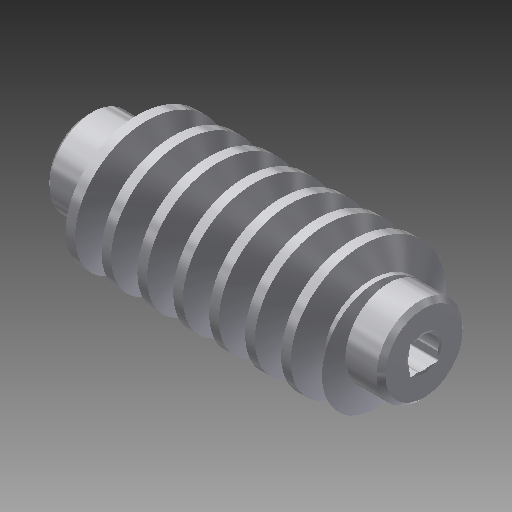
# Autodesk Inventor part: 400-04
Saved by Autodesk Inventor 2019 (Build 230136000, 136)
## iProperties
Created: 2007-11-19
Part Number: 400-04
Material: Acetal Resin, White
Document SubType Name: Modeling
Designer: Autodesk Inc.
Density: 1.425 g/cm^3
Mass: 5.8548 g
Surface Area: 32.563 cm^2
Volume: 4.10863 cm^3
Description: WORM GEAR
Appearance: Smooth - White
CustomPartVersion: 1
Company: Autodesk Inc.
Component Category: Lower Component
d49: 20.000 mm
d50: 0.000 mm
d54: 0.000 mm
d56: 0.000 mm
d77: 0.000 mm
d79: 20.000 mm
d80: 0.000 mm
Author: Inventor
Autodesk Inventor part; units mm, degrees
ref_plane "YZ Plane" through (0, 0, 0) normal (1, 0, 0) x (0, 1, 0)
ref_plane "XZ Plane" through (0, 0, 0) normal (0, 1, 0) x (-1, 0, 0)
ref_plane "XY Plane" through (0, 0, 0) normal (0, 0, 1) x (1, 0, 0)
sketch "Base Body Sketch" plane through (0, 0, 0) normal (1, 0, 0) x (0, 1, 0)
  circle A0 centre (0, 0) radius 7.761668
  dimension "d5" = 15.52334
extrude "Base Body" add sketch "Base Body Sketch" along normal mid plane 30
sketch "Sketch5" plane through (15, 0, 0) normal (1, 0, 0) x (0, 0, -1)
  circle A0 centre (0, 0) radius 7.761668
  circle A1 centre (0, 0) radius 6.5
  dimension "d59" = 13
  constraints: 1 centre point, 1 coincident
  measures "d59" diameter of A1
sketch "Sketch7" plane through (0, 0, 0) normal (0, 1, 0) x (-1, 0, 0)
  line L0 (13.658997, -4.915723) -> (12.757003, -4.915723)
  line L1 (11.721164, -7.761668) -> (10.630836, -7.761668)
  line L2 (9.594997, -4.915723) -> (8.693003, -4.915723)
  line L3 (7.657164, -7.761668) -> (6.566836, -7.761668)
  line L4 (5.530997, -4.915723) -> (4.629003, -4.915723)
  line L5 (3.593164, -7.761668) -> (2.502836, -7.761668)
  line L6 (1.466997, -4.915723) -> (0.565003, -4.915723)
  line L7 (-0.470836, -7.761668) -> (-1.561164, -7.761668)
  line L8 (-2.597003, -4.915723) -> (-3.498997, -4.915723)
  line L9 (15, 4.915723) -> (15, 4.865723)
  line L10 (15, 4.865723) -> (18.5, 4.865723)
  line L11 (18.5, 4.865723) -> (19, 4.365723)
  line L12 (19, 4.365723) -> (19, -4.365723)
  line L13 (19, -4.365723) -> (18.5, -4.865723)
  line L14 (18.5, -4.865723) -> (15, -4.865723)
  line L15 (15, -4.865723) -> (15, -4.915723)
  line L16 (19, 0) -> (27, 0) construction
  arc A0 (19, 2.015564) -> (18.75, 0) centre (27, 0) ccw
  line L17 (19, 0) -> (18.75, 0)
  line L18 (19, 0) -> (19, 2.015564)
  line L19 (15, -4.915723) -> (14.329498, -6.757911)
  line L20 (-15, 4.915723) -> (-14.329498, 6.757911)
  line L21 (-4.534836, -7.761668) -> (-5.625164, -7.761668)
  line L22 (-11.721164, 7.761668) -> (-10.630836, 7.761668)
  line L23 (-13.658997, 4.915723) -> (-12.757003, 4.915723)
  line L24 (-7.657164, 7.761668) -> (-6.566836, 7.761668)
  line L25 (-9.594997, 4.915723) -> (-8.693003, 4.915723)
  line L26 (14.789003, 4.915723) -> (15, 4.915723)
  line L27 (-6.661003, -4.915723) -> (-7.562997, -4.915723)
  line L28 (-8.598836, -7.761668) -> (-9.689164, -7.761668)
  line L29 (-10.725003, -4.915723) -> (-11.626997, -4.915723)
  line L30 (-12.662836, -7.761668) -> (-13.753164, -7.761668)
  line L31 (-14.789003, -4.915723) -> (-15, -4.915723)
  line L32 (-15, -4.915723) -> (-15, 4.915723)
  line L33 (-5.530997, 4.915723) -> (-4.629003, 4.915723)
  line L34 (-3.593164, 7.761668) -> (-2.502836, 7.761668)
  line L35 (-1.466997, 4.915723) -> (-0.565003, 4.915723)
  line L36 (0.470836, 7.761668) -> (1.561164, 7.761668)
  line L37 (2.597003, 4.915723) -> (3.498997, 4.915723)
  line L38 (4.534836, 7.761668) -> (5.625164, 7.761668)
  line L39 (6.661003, 4.915723) -> (7.562997, 4.915723)
  line L40 (8.598836, 7.761668) -> (9.689164, 7.761668)
  line L41 (10.725003, 4.915723) -> (11.626997, 4.915723)
  line L42 (12.662836, 7.761668) -> (13.753164, 7.761668)
  dimension "d87" = 8
  dimension "d88" = 16.5
  constraints: 6 end point, 2 collinear, 2 point on circle, 1 centre point, 1 coincident, 1 midpoint, 1 perpendicular, 1 point on line, 30 other
  measures "d87" distance of L16.start L16.end
  measures "d88" diameter of A0
surface extrude "ExtrusionSrf1" sketch "Sketch5" against normal through all shown no curves A1
chamfer "Chamfer1" distance 1.035839 distance2 2.845945 1 edges at (15, -7.7617, 0) measured on face at (10, 7.7365, -0.6246)
chamfer "Chamfer2" distance 1.035839 distance2 2.845945 1 edges at (-15, -7.7617, 0) measured on face at (-10, 7.7365, -0.6246)
sketch "Tooth Sketch" plane through (0, 0, 0) normal (0, 0, 1) x (1, 0, 0)
  line L0 (0, 8.423997) -> (0, 4.331011)
  line L1 (-19.803086, 7.839285) -> (-18.738997, 4.915723)
  line L2 (-17.837003, 4.915723) -> (-16.772914, 7.839285)
  line L3 (-20.409121, 0) -> (-16.166879, 0)
  line L4 (-19.803086, 7.839285) -> (-18.288, 7.839285)
  line L5 (-18.288, 7.839285) -> (-16.772914, 7.839285)
  line L6 (-18.738997, 4.915723) -> (-18.288, 4.915723)
  line L7 (-18.288, 4.915723) -> (-17.837003, 4.915723)
  line L8 (-18.288, 6.468057) -> (-17.272, 6.468057) construction
  line L9 (-18.288, 7.839285) -> (-18.288, 4.915723) construction
  dimension "d24" = 110
  dimension "d25" = 18.288
  dimension "d26" = 1.016
  dimension "d27" = 4.91572
  dimension "d28" = 6.46806
  dimension "d29" = 7.83928
  constraints: 16 end point, 3 equal length, 3 parallel, 2 collinear, 2 point on line
  measures "d24" angle of L6 L1
  measures "d25" distance from line of L0 L4.end
  measures "d26" distance of L8.start L8.end
  measures "d27" distance between parallel lines of L3 L6
  measures "d28" distance between parallel lines of L3 L8
  measures "d29" distance between parallel lines of L3 L4
feature "Tooth" [suppressed]
pattern_circular "Tooth Pattern" [suppressed]
coil "Left Tooth" sketch "Tooth Sketch" operation cut axis through (-10, 0, 0) along (1, 0, 0) pitch 4.064 turns 10 hand left
pattern_of_one "Left Tooth Pattern"
sketch "Sketch6" plane through (-15, 0, 0) normal (-1, 0, 0) x (0, 0, 1)
  arc A0 (4.65648, -1.575285) -> (2.36739, 4.308109) centre (0, 0) ccw
  circle A1 centre (0, 0) radius 4.865723
  arc A2 (2.36739, 4.308109) -> (4.65648, -1.575285) centre (0, 0) ccw
  dimension "d83" = 0.05
  constraints: 1 centre point, 1 coincident
  measures "d83" radial gap between concentric circles of A2 A1
sketch "Sketch6 outline for Extrusion2" plane through (-15, 0, 0) normal (-1, 0, 0) x (0, 0, 1)
  circle A0 centre (0, 0) radius 4.865723
extrude "Extrusion2" add sketch "Sketch6 outline for Extrusion2" along normal blind 4
chamfer "Chamfer3" distance 0.5 angle 45 1 edges at (-19, 0, -4.8657)
revolve "Revolution1" cut sketch "Sketch7" angle 360 about axis through (-19, 0, 0) along (-1, 0, 0)
mirror "Mirror1" about plane through (0, 0, 0) normal (1, 0, 0) of "Extrusion2", "Chamfer3", "Revolution1"
sketch "Sketch8" plane through (-19, 0, 0) normal (-1, 0, 0) x (0, 0, 1)
  circle A0 centre (0, 0) radius 2.015564
  line L0 (-1.625, 1.625) -> (1.625, 1.625)
  line L1 (1.625, 1.625) -> (1.625, -1.625)
  line L2 (1.625, -1.625) -> (-1.625, -1.625)
  line L3 (-1.625, -1.625) -> (-1.625, 1.625)
  circle A1 centre (0, 0) radius 4.365723
  circle A2 centre (0, 0) radius 1.75
  dimension "d90" = 3.25
  dimension "d91" = 3.25
  dimension "d92" = 1.625
  dimension "d93" = 1.625
  dimension "d96" = 3.5
  constraints: 8 end point, 2 parallel, 1 centre point, 1 coincident, 1 horizontal, 1 perpendicular
  measures "d90" distance of L0.start L0.end
  measures "d91" distance of L0.end L1.end
  measures "d92" distance from line of L0 A0.centre
  measures "d93" distance from line of L3 A0.centre
  measures "d96" diameter of A2
sketch "Sketch8 outline for Extrusion3" plane through (-19, 0, 0) normal (-1, 0, 0) x (0, 0, 1)
  line L0 (-1.625, 1.625) -> (-0.649519, 1.625)
  line L1 (-1.625, 0.649519) -> (-1.625, 1.625)
  arc A0 (-1.625, 0.649519) -> (-1.625, -0.649519) centre (0, 0) ccw
  line L2 (-1.625, -1.625) -> (-1.625, -0.649519)
  line L3 (-0.649519, -1.625) -> (-1.625, -1.625)
  arc A1 (-0.649519, -1.625) -> (0.649519, -1.625) centre (0, 0) ccw
  line L4 (1.625, -1.625) -> (0.649519, -1.625)
  line L5 (1.625, -0.649519) -> (1.625, -1.625)
  arc A2 (1.625, -0.649519) -> (1.625, 0.649519) centre (0, 0) ccw
  line L6 (1.625, 1.625) -> (1.625, 0.649519)
  line L7 (0.649519, 1.625) -> (1.625, 1.625)
  arc A3 (0.649519, 1.625) -> (-0.649519, 1.625) centre (0, 0) ccw
extrude "Extrusion3" cut sketch "Sketch8 outline for Extrusion3" against normal through all
fillet "Fillet1" radius 0.2 4 edges at (0, -1.625, -1.625) (0, -1.625, 1.625) (0, 1.625, -1.625) (0, 1.625, 1.625)
equation "\"d6\" = da_b"
equation "\"d8\" = fd_cham1"
equation "\"d9\" = 0.5 * fd_cham2"
equation "\"d10\" = fd_cham1"
equation "\"d11\" = 0.5 * fd_cham2"
equation "\"d25\" = fd_dist"
equation "\"d26\" = 0.25 * da_px"
equation "\"d27\" = 0.5 * da_df"
equation "\"d28\" = 0.5 * da_d"
equation "\"d29\" = 0.505 * da_da"
equation "\"d32\" = fd_n"
equation "\"da_rightdir\" = 0"
equation "\"d64\" = fd_n"
equation "\"d90\" = d91"
equation "\"d92\" = 0.5 * d91"
equation "\"d93\" = 0.5 * d90"
equation "\"d5\" = da_da"
equation "\"da_b\" = 30"
equation "\"da_df\" = 9.83145"
equation "\"da_da\" = 15.52334"
equation "\"fd_cham2\" = da_da - da_df"
equation "\"fd_cham1\" = 0.181985 * fd_cham2"
equation "\"da_d\" = 12.93611"
equation "\"da_px\" = 4.064"
equation "\"da_alfat\" = 20deg"
equation "\"d49\" = da_aw"
equation "\"d79\" = da_aw"
equation "\"fd_dist\" = 18.288"
equation "\"fd_n\" = 10"
equation "\"da_aw\" = 20"
body "Solid1"
body "Srf1"
